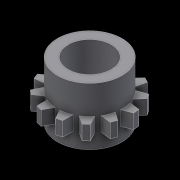
# Autodesk Inventor part: ChainGear
Saved by Autodesk Inventor 2015 (Build 190159000, 159)
## iProperties
Created: 2015-07-30
Part Number: ChainGear
Material: Generic
Document SubType Name: Modeling
Designer: Val
Density: 1 g/cm^3
Appearance: Default
Author: Val
Autodesk Inventor part; units mm, degrees
ref_plane "YZ Plane" through (0, 0, 0) normal (1, 0, 0) x (0, 1, 0)
ref_plane "XZ Plane" through (0, 0, 0) normal (0, 1, 0) x (-1, 0, 0)
ref_plane "XY Plane" through (0, 0, 0) normal (0, 0, 1) x (1, 0, 0)
sketch "Sketch1" plane through (0, 0, 0) normal (0, 0, 1) x (1, 0, 0)
  circle A0 centre (0, 0) radius 3
  circle A1 centre (0, 0) radius 1.5
  dimension "d0" = 6
  dimension "d1" = 3
  constraints: 2 centre point, 2 coincident
  measures "d0" diameter of A0
  measures "d1" diameter of A1
extrude "Extrusion1" add sketch "Sketch1" along normal blind 1
sketch "Sketch3" plane through (0, 0, 0) normal (0, 0, -1) x (-1, 0, 0)
  circle A0 centre (0, 0) radius 1.5 projected
  circle A1 centre (0, 0) radius 3 projected
extrude "Extrusion3" add sketch "Sketch3" along normal blind 1
sketch "Sketch2" plane through (0, 0, 1) normal (0, 0, 1) x (1, 0, 0)
  line L0 (0, 0) -> (0, 3.959) construction
  line L1 (-0.15, 3.959) -> (0.15, 3.959)
  line L2 (-0.4943, 2.959) -> (0.4943, 2.959)
  line L3 (-0.15, 3.959) -> (-0.4943, 2.959)
  line L4 (0.15, 3.959) -> (0.4943, 2.959)
  circle A0 centre (0, 0) radius 3 projected
  point P0 (0, 2.959)
  dimension "d4" = 1
  dimension "d5" = 0.3
  dimension "d8" = 109
  constraints: 10 end point, 2 horizontal, 2 midpoint, 1 point on line, 1 vertical, 2 other
  measures "d4" distance between parallel lines of L1 L2
  measures "d5" distance of L1.start L1.end
  measures "d8" angle of L3 L1
extrude "Extrusion2" add sketch "Sketch2" against normal up to surface (1 mm away) separate body contours L1 L4 A0 L3 | A0 L2 picked at (-0.0551, 2.9711)
sketch "Sketch4" plane through (0, 0, 1) normal (0, 0, 1) x (1, 0, 0)
  circle A0 centre (0, 0) radius 1.5 projected
  circle A1 centre (0, 0) radius 3 projected
extrude "Extrusion4" add sketch "Sketch4" along normal blind 4 bodies 1
pattern_circular "Circular Pattern1" count 9 over 360 about axis through (0, 0, 0) along (0, 0, 1) of "Extrusion2" bodies 2
combine bodies "Combine1" operation type add bodies to combine 1 2
body "Solid2"
